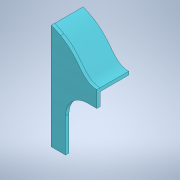
# Autodesk Inventor part: obudowa przekładni 6 RIGHT
Saved by Autodesk Inventor 2021 (Build 250183000, 183)
## iProperties
Created: 2022-01-26
Part Number: obudowa przekładni 6 RIGHT
Material: Generic
Document SubType Name: Modeling
Designer: Łukasz
Density: 1 g/cm^3
Appearance: Cadet Blue
Author: Łukasz
Autodesk Inventor part; units mm, degrees
ref_plane "YZ Plane" through (0, 0, 0) normal (1, 0, 0) x (0, 1, 0)
ref_plane "XZ Plane" through (0, 0, 0) normal (0, 1, 0) x (-1, 0, 0)
ref_plane "XY Plane" through (0, 0, 0) normal (0, 0, 1) x (1, 0, 0)
sketch "Sketch1" plane through (0, 0, 0) normal (0, 0, 1) x (1, 0, 0)
  line L0 (0, 0) -> (-13, 0)
  line L1 (-13, 0) -> (-13, 92)
  line L2 (-13, 92) -> (0, 92)
  line L3 (0, 92) -> (0, 0)
  dimension "d0" = 13
  dimension "d1" = 92
  constraints: 8 end point, 2 parallel, 1 horizontal, 1 perpendicular
  measures "d0" distance of L1.end L2.end
  measures "d1" distance of L0.end L1.end
extrude "Extrusion1" add sketch "Sketch1" along normal blind 3
sketch "Sketch3" plane through (0, 0, 3) normal (0, 0, 1) x (1, 0, 0)
  line L0 (0, 92) -> (-13, 92) projected
  line L1 (0, 92) -> (28.5, 92)
  line L2 (28.5, 92) -> (28.5, 51)
  line L3 (28.5, 51) -> (0, 51)
  line L4 (0, 51) -> (0, 92)
  point P0 (0, 0)
  dimension "d6" = 28.5
  dimension "d7" = 41
  constraints: 8 end point, 2 parallel, 1 horizontal, 1 perpendicular
  measures "d6" distance of L2.end L3.end
  measures "d7" distance of L1.end L2.end
extrude "Extrusion3" add sketch "Sketch3" against normal up to surface (3 mm away)
sketch "Sketch4" plane through (0, 0, 0) normal (0, 0, -1) x (-1, 0, 0)
  arc A0 (40, 102.8631) -> (0, 62.8631) centre (40, 62.8631) ccw
  arc A1 (-28.5, 65.8631) -> (-42.9914, -4.1369) centre (-28.5, 29.3631) ccw
  line L0 (13, 92) -> (0, 92)
  line L1 (0, 92) -> (-28.5, 92)
  line L2 (-28.5, 92) -> (-28.5, 51)
  line L3 (-28.5, 92) -> (13, 92) projected
  line L4 (-28.5, 65.8631) -> (-28.5, 62.8631)
  line L5 (-28.5, 51) -> (-28.5, 92) projected
  line L6 (13, 92) -> (13, 89)
  line L7 (13, 92) -> (13, 0) projected
  arc A2 (40, 105.4873) -> (13, 95.9537) centre (40, 62.4873) ccw
  line L8 (13, 92) -> (13, 95.9537)
  line L9 (13, 92) -> (-10.5212, 84.6591) construction
  line L10 (-10.5212, 84.6591) -> (-7.75, 64.3631) construction
  line L11 (-7.75, 64.3631) -> (-28.5, 62.8631) construction
  spline S0 degree 3 poles (13, 92) (-10.5212, 84.6591) (-7.75, 64.3631) (-28.5, 62.8631) knots 1 1 1 1 2 2 2 2
  line L12 (13, 95.9537) -> (-14.25, 85.7047) construction
  line L13 (-14.25, 85.7047) -> (-11.7162, 66.3603) construction
  line L14 (-11.7162, 66.3603) -> (-28.5, 65.8631) construction
  spline S1 degree 3 poles (13, 95.9537) (-14.25, 85.7047) (-11.7162, 66.3603) (-28.5, 65.8631) knots 1 1 1 1 2 2 2 2
  point P0 (0, 0)
  point P1 (12.3882, 91.8042)
  point P2 (13, 92.3758)
  dimension "d10" = 3
  dimension "d11" = 3
  constraints: 12 end point, 6 point on circle, 3 centre point, 2 point on line, 6 other
  measures "d10" distance of L4.start L4.end
  measures "d11" distance of L3.end L6.end
extrude "Extrusion4" add sketch "Sketch4" along normal blind 26 contours A0 L0 S1 L8 | A0 S0 L2 S1 L0
sketch "Sketch5" plane through (0, 0, 0) normal (0, 0, -1) x (-1, 0, 0)
  spline S0 degree 3 poles (-28.5, 65.8631) (-13.6927, 66.3017) (-13.9211, 81.4099) (4.5317, 92) knots 0 0 0 0 1 1 1 1 projected
  line L0 (-28.5, 92) -> (4.5317, 92) projected
  line L1 (-28.5, 92) -> (-28.5, 65.8631) projected
  point P0 (0, 0)
  constraints: 1 other
extrude "Extrusion5" cut sketch "Sketch5" against normal blind 40
sketch "Sketch6" plane through (0, 0, 0) normal (0, 0, 1) x (1, 0, 0)
  line L0 (-4.5317, 92) -> (-12.5949, 92) projected
  spline S0 degree 3 poles (-13, 95.9537) (-9.7909, 94.7467) (-6.9949, 93.4136) (-4.5317, 92) knots 0 0 0 0 1 1 1 1 projected
  line L1 (-13, 92.3758) -> (-13, 95.9537) projected
  arc A0 (-12.5949, 92) -> (-13, 92.3758) centre (-40, 62.8631) ccw projected
  arc A1 (-12.5949, 92) -> (-13, 92.3758) centre (-40, 62.8631) ccw projected
  line L2 (-13, 92.3758) -> (-13, 92)
  line L3 (-13, 92) -> (-12.5949, 92)
  point P0 (0, 0)
  constraints: 4 end point, 1 vertical, 1 other
extrude "Extrusion6" add sketch "Sketch6" along normal up to surface (3 mm away)
sketch "Sketch7" plane through (0, 0, -26) normal (0, 0, -1) x (-1, 0, 0)
  spline S0 degree 3 poles (-28.5, 62.8631) (-7.9317, 64.3502) (-10.4747, 84.3054) (12.3882, 91.8042) knots 1 1 1 1 1.991245 1.991245 1.991245 1.991245
  arc A0 (40, 102.8631) -> (0, 62.8631) centre (40, 62.8631) ccw
  line L0 (0, 62.8631) -> (-28.5, 62.8631)
  line L1 (-28.5, 62.8631) -> (-28.5, 65.8631)
  line L2 (-28.5, 51) -> (-28.5, 65.8631) projected
  point P0 (0, 0)
  constraints: 4 end point, 2 point on circle, 1 centre point, 3 other
extrude "Extrusion7" add sketch "Sketch7" against normal blind 3
fillet "Fillet1" radius 20 1 edges at (0, 51, 1.5)
body "Solid1"
